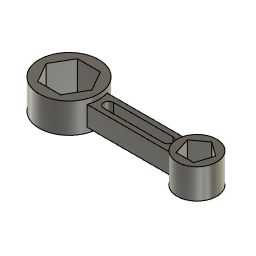
Exercise_02 (Autodesk Fusion 360 design; units mm, degrees)
Autodesk Fusion 360 part; units mm, degrees
sketch "Sketch1" plane through (0, 0, 0) normal (0, 0, 1) x (1, 0, 0)
  circle A0 centre (-75, 0) radius 30
  circle A1 centre (54, 0) radius 20
  line L0 (-86.547, 20) -> (-98.094, 0)
  line L1 (-98.094, 0) -> (-86.547, -20)
  line L2 (-86.547, -20) -> (-63.453, -20)
  line L3 (-63.453, -20) -> (-51.906, 0)
  line L4 (-51.906, 0) -> (-63.453, 20)
  line L5 (-63.453, 20) -> (-86.547, 20)
  line L6 (54, 15) -> (39.7342, 4.6353)
  line L7 (39.7342, 4.6353) -> (45.1832, -12.1353)
  line L8 (45.1832, -12.1353) -> (62.8168, -12.1353)
  line L9 (62.8168, -12.1353) -> (68.2658, 4.6353)
  line L10 (68.2658, 4.6353) -> (54, 15)
  line L11 (-46.7157, 10) -> (36.6795, 10)
  line L12 (-46.7157, -10) -> (36.6795, -10)
  line L13 (-35, 5) -> (25, 5)
  line L14 (25, -5) -> (-35, -5)
  arc A2 (25, -5) -> (25, 5) centre (25, 0) ccw
  line L15 (-75, 0) -> (-40, 0)
  line L16 (30, 0) -> (54, 0)
  arc A3 (-35, 5) -> (-35, -5) centre (-35, 0) ccw
  point P0 (-75, 0)
  point P1 (54, 0)
  dimension "d1" = 60
  dimension "d2" = 129
  dimension "d3" = 40
  dimension "d4" = 20
  dimension "d5" = 15
  dimension "d6" = 10
  dimension "d7" = 10
  constraint coincident P0 A0.centre
  constraint horizontal L15
  constraint coincident P1 A1.centre
  constraint coincident A1 L11.end
  constraint horizontal L11
  constraint horizontal L12
  constraint coincident A1 L12.end
  constraint coincident A0 L11.start
  constraint coincident A0 L12.start
  constraint horizontal L13
  constraint horizontal L14
  constraint coincident A3.centre L15
  constraint tangent L13 A3
  constraint coincident A2.centre L15
  constraint tangent L13 A2
  constraint coincident A2 L16.start
  constraint collinear L15 L16
  measures "d1" diameter of A0
  measures "d2" distance of P0 P1
  measures "d3" diameter of A1
  measures "d4" distance of P0 L5
  measures "d5" distance of L6.start P1
  measures "d6" distance of L11 L15
  measures "d7" distance of L12 L15
extrude "Extrude1" add sketch "Sketch1" along normal mid plane 30 contours A0 | A1 makes body 1 at (-47.8338, -12.7278, 5) makes body 2 at (73.9006, -1.9914, -5)
extrude "Extrude2" add sketch "Sketch1" along normal mid plane 20 contours A0 A1 L12 L14 A2 L15 L16 A3 | A0 A1 L11 L13 A2 L15 L16 A3 bodies 1 2
